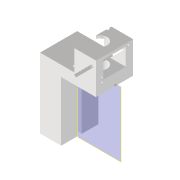
# Autodesk Inventor part: 30_XYTabel_Aliexpress_cellSTORM_lasermount
Saved by Autodesk Inventor 2022 (Build 260153000, 153)
## iProperties
Created: 2021-12-30
Part Number: 30_XYTabel_Aliexpress_cellSTORM_lasermount
Material: Generisch
Document SubType Name: Modeling
Designer: diederichbenedict
Density: 1 g/cm^3
Appearance: Vorgabe
Author: diederichbenedict
Autodesk Inventor part; units mm, degrees
ref_plane "YZ Plane" through (0, 0, 0) normal (1, 0, 0) x (0, 1, 0)
ref_plane "XZ Plane" through (0, 0, 0) normal (0, 1, 0) x (-1, 0, 0)
ref_plane "XY Plane" through (0, 0, 0) normal (0, 0, 1) x (1, 0, 0)
ref_plane "Arbeitsebene1" through (-8.5351, 221.2503, 0) normal (0, 0, -1) x (0, 1, 0)
sketch "Skizze1" plane through (-8.5351, 221.2503, 0) normal (0, 0, -1) x (0, 1, 0)
  circle A0 centre (33, 16) radius 1.4 projected
  circle A1 centre (33, 8) radius 1.4 projected
  circle A2 centre (33, 24) radius 1.4 projected
  circle A3 centre (5, 16) radius 1.4 projected
  circle A4 centre (5, 8) radius 1.4 projected
  circle A5 centre (5, 24) radius 1.4 projected
  circle A6 centre (43, 8) radius 1.4 projected
  circle A7 centre (43, 16) radius 1.4 projected
  circle A8 centre (43, 24) radius 1.4 projected
  line L0 (0, 32) -> (0, 0) projected
  line L1 (0, 32) -> (48, 32) projected
  line L2 (48, 0) -> (48, 32) projected
  line L3 (0, 0) -> (48, 0) projected
  arc A9 (65.2166, -9.3098) -> (65.4479, -9.4649) centre (65.4479, -9.2149) ccw projected
  arc A10 (65.2166, -9.3098) -> (64.7173, -8.7321) centre (64.1062, -9.7649) ccw projected
  arc A11 (64.5955, -8.5388) -> (64.7173, -8.7321) centre (64.8445, -8.517) ccw projected
  line L4 (64.5955, -8.5388) -> (64.5653, -8.1931) projected
  arc A12 (64.5653, -8.1931) -> (64.3162, -7.9649) centre (64.3162, -8.2149) ccw projected
  line L5 (64.3162, -7.9649) -> (63.8638, -7.9649) projected
  arc A13 (63.8638, -7.9649) -> (63.6147, -8.1931) centre (63.8638, -8.2149) ccw projected
  line L6 (63.6147, -8.1931) -> (63.5827, -8.5597) projected
  arc A14 (63.4668, -8.7495) -> (63.5827, -8.5597) centre (63.3336, -8.5379) ccw projected
  arc A15 (63.4668, -8.7495) -> (62.9959, -9.3098) centre (64.1062, -9.7649) ccw projected
  arc A16 (62.7646, -9.4649) -> (62.9959, -9.3098) centre (62.7646, -9.2149) ccw projected
  line L7 (62.7646, -9.4649) -> (62.09, -9.4649) projected
  line L8 (62.09, -9.4649) -> (61.59, -8.9649) projected
  line L9 (61.59, -8.9649) -> (61.59, 2.0351) projected
  line L10 (61.59, 2.0351) -> (62.09, 2.5351) projected
  line L11 (62.09, 2.5351) -> (62.7646, 2.5351) projected
  arc A17 (62.9959, 2.3799) -> (62.7646, 2.5351) centre (62.7646, 2.2851) ccw projected
  arc A18 (62.9959, 2.3799) -> (63.4668, 1.8196) centre (64.1062, 2.8351) ccw projected
  arc A19 (63.5827, 1.6298) -> (63.4668, 1.8196) centre (63.3336, 1.608) ccw projected
  line L12 (63.5827, 1.6298) -> (63.6147, 1.2633) projected
  arc A20 (63.6147, 1.2633) -> (63.8638, 1.0351) centre (63.8638, 1.2851) ccw projected
  line L13 (63.8638, 1.0351) -> (64.3162, 1.0351) projected
  arc A21 (64.3162, 1.0351) -> (64.5653, 1.2633) centre (64.3162, 1.2851) ccw projected
  line L14 (64.5653, 1.2633) -> (64.5955, 1.6089) projected
  arc A22 (64.7173, 1.8023) -> (64.5955, 1.6089) centre (64.8445, 1.5871) ccw projected
  arc A23 (64.7173, 1.8023) -> (65.2166, 2.3799) centre (64.1062, 2.8351) ccw projected
  arc A24 (65.4479, 2.5351) -> (65.2166, 2.3799) centre (65.4479, 2.2851) ccw projected
  line L15 (65.4479, 2.5351) -> (66.59, 2.5351) projected
  line L16 (66.59, 2.5351) -> (66.59, 9.1351) projected
  line L17 (66.59, 9.1351) -> (65.99, 9.7351) projected
  line L18 (65.99, 9.7351) -> (58.19, 9.7351) projected
  line L19 (58.19, 9.7351) -> (56.99, 8.5351) projected
  line L20 (56.99, 8.5351) -> (56.99, -15.4649) projected
  line L21 (56.99, -15.4649) -> (58.19, -16.6649) projected
  line L22 (58.19, -16.6649) -> (65.99, -16.6649) projected
  line L23 (65.99, -16.6649) -> (66.59, -16.0649) projected
  line L24 (66.59, -16.0649) -> (66.59, -9.4649) projected
  line L25 (66.59, -9.4649) -> (65.4479, -9.4649) projected
  circle A25 centre (59.585, 3.4351) radius 2.1 projected
  circle A26 centre (59.585, -10.3649) radius 2.1 projected
  line L26 (56.59, 2.9351) -> (56.59, 9.435) projected
  line L27 (56.99, 2.5351) -> (56.59, 2.9351) projected
  arc A27 (64.7172, 1.8023) -> (65.2166, 2.3799) centre (64.1062, 2.8351) ccw projected
  arc A28 (65.4479, 2.5351) -> (65.2166, 2.3799) centre (65.4479, 2.2851) ccw projected
  line L28 (66.59, 2.5351) -> (65.4479, 2.5351) projected
  line L29 (66.59, 9.4351) -> (66.59, 2.5351) projected
  line L30 (65.99, 10.0351) -> (66.59, 9.4351) projected
  line L31 (57.19, 10.0351) -> (65.99, 10.0351) projected
  line L32 (56.59, 9.435) -> (57.19, 10.0351) projected
  line L33 (56.59, 2.9351) -> (56.59, 9.435) projected
  line L34 (56.99, 2.5351) -> (56.59, 2.9351) projected
  line L35 (56.99, -9.4649) -> (56.99, 2.5351) projected
  line L36 (56.59, -9.8649) -> (56.99, -9.4649) projected
  line L37 (56.59, -16.3649) -> (56.59, -9.8649) projected
  line L38 (57.19, -16.9649) -> (56.59, -16.3649) projected
  line L39 (61.79, -16.9649) -> (57.19, -16.9649) projected
  arc A29 (62.59, -16.9649) -> (61.79, -16.9649) centre (62.19, -17.2649) ccw projected
  line L40 (65.99, -16.9649) -> (62.59, -16.9649) projected
  line L41 (66.59, -16.3649) -> (65.99, -16.9649) projected
  line L42 (66.59, -9.4649) -> (66.59, -16.3649) projected
  line L43 (65.4479, -9.4649) -> (66.59, -9.4649) projected
  arc A30 (65.2166, -9.3098) -> (65.4479, -9.4649) centre (65.4479, -9.2149) ccw projected
  arc A31 (65.2166, -9.3098) -> (64.7172, -8.7321) centre (64.1062, -9.7649) ccw projected
  arc A32 (64.5955, -8.5388) -> (64.7172, -8.7321) centre (64.8445, -8.517) ccw projected
  line L44 (64.5653, -8.1931) -> (64.5955, -8.5388) projected
  arc A33 (64.5653, -8.1931) -> (64.3162, -7.9649) centre (64.3162, -8.2149) ccw projected
  line L45 (63.8638, -7.9649) -> (64.3162, -7.9649) projected
  arc A34 (63.8638, -7.9649) -> (63.6147, -8.1931) centre (63.8638, -8.2149) ccw projected
  line L46 (63.5827, -8.5597) -> (63.6147, -8.1931) projected
  arc A35 (63.4668, -8.7495) -> (63.5827, -8.5597) centre (63.3336, -8.5379) ccw projected
  arc A36 (63.4668, -8.7495) -> (62.9959, -9.3098) centre (64.1062, -9.7649) ccw projected
  arc A37 (62.7646, -9.4649) -> (62.9959, -9.3098) centre (62.7646, -9.2149) ccw projected
  line L47 (62.09, -9.4649) -> (62.7646, -9.4649) projected
  line L48 (61.59, -8.9649) -> (62.09, -9.4649) projected
  line L49 (61.59, 2.0351) -> (61.59, -8.9649) projected
  line L50 (62.09, 2.5351) -> (61.59, 2.0351) projected
  line L51 (62.7646, 2.5351) -> (62.09, 2.5351) projected
  arc A38 (62.9959, 2.3799) -> (62.7646, 2.5351) centre (62.7646, 2.2851) ccw projected
  arc A39 (62.9959, 2.3799) -> (63.4668, 1.8196) centre (64.1062, 2.8351) ccw projected
  arc A40 (63.5827, 1.6298) -> (63.4668, 1.8196) centre (63.3336, 1.6081) ccw projected
  line L52 (63.6147, 1.2633) -> (63.5827, 1.6298) projected
  arc A41 (63.6147, 1.2633) -> (63.8638, 1.0351) centre (63.8638, 1.2851) ccw projected
  line L53 (64.3162, 1.0351) -> (63.8638, 1.0351) projected
  arc A42 (64.3162, 1.0351) -> (64.5653, 1.2633) centre (64.3162, 1.2851) ccw projected
  line L54 (64.5955, 1.6089) -> (64.5653, 1.2633) projected
  arc A43 (64.7172, 1.8023) -> (64.5955, 1.6089) centre (64.8445, 1.5871) ccw projected
  line L55 (85.0966, 28.1351) -> (41.8486, 28.1351)
  line L56 (61.6219, 29.1351) -> (61.6219, 34.6351)
  line L57 (66.9191, 29.1351) -> (66.9191, 34.6351)
  line L58 (0, 0) -> (56.64, 0)
  line L59 (56.64, 0) -> (56.64, -17.0149)
  line L60 (56.64, -17.0149) -> (0, -17.0149)
  line L61 (0, -17.0149) -> (0, 0)
  line L62 (56.64, 0) -> (48, 0)
  line L63 (48, 0) -> (48, 28.1351)
  line L64 (48, 28.1351) -> (56.64, 28.1351)
  line L65 (56.64, 28.1351) -> (56.64, 0)
  line L66 (73.5914, 28.1351) -> (56.64, 28.1351)
  line L67 (56.64, 28.1351) -> (56.64, 10.5351)
  line L68 (56.64, 10.5351) -> (73.5914, 10.5351)
  line L69 (73.5914, 10.5351) -> (73.5914, 28.1351)
  line L70 (73.59, 15.5051) -> (73.59, -22.4349)
  line L71 (73.59, 15.5051) -> (73.59, -22.4349)
  point P0 (-221.2503, 8.5351)
  point P1 (56.64, -16.4149)
  point P2 (56.64, -9.8149)
  point P3 (56.64, 2.8851)
  point P4 (56.64, 9.4851)
  dimension "d0" = 0.5
  constraints: 34 end point, 6 parallel, 4 horizontal, 4 vertical, 3 perpendicular, 3 point on line, 10 other
  measures "d0" distance between parallel lines of L68 L31
extrude "Extrusion1" add sketch "Skizze1" along normal mid plane 30 contours L3 L58 L59 L36 L37 L38 L60 L61 | L2 L55 L65 L32 L26 L27 L58 | L55 L69 L68 L65
sketch "Skizze2" plane through (-25.55, 221.2503, -15) normal (-1, 0, 0) x (0, 0, 1)
  circle A0 centre (15, 5) radius 1.4 projected
  circle A1 centre (15, 33) radius 1.4 projected
  line L0 (15, 33) -> (15, 0) construction
  line L1 (30, 0) -> (0, 0) projected
  line L2 (13.4, 33) -> (13.4, 0)
  line L3 (16.6, 0) -> (16.6, 33)
  arc A2 (16.6, 33) -> (13.4, 33) centre (15, 33) ccw
  arc A3 (13.4, 0) -> (16.6, 0) centre (15, 0) ccw
  point P0 (15, -221.2503)
  point P1 (15, 16.5)
  dimension "d3" = 3.2
  constraints: 8 end point, 4 point on circle, 4 tangent, 2 centre point, 2 midpoint, 1 parallel
  measures "d3" diameter of A3
extrude "Extrusion2" cut sketch "Skizze2" against normal blind 30 contours A0 | A1 | A3 L1 | L1 L2 A2 L3
sketch "Skizze3" plane through (19.6, 269.2503, -15) normal (1, 0, 0) x (0, 0, -1)
  arc A0 (0.8555, 0.89) -> (1.8555, -0.11) centre (1.8555, 0.89) ccw projected
  line L0 (1.8555, -0.11) -> (5, -0.11) projected
  line L1 (5, -0.11) -> (5, 25.59) projected
  line L2 (5, 25.59) -> (-4.5277, 25.59) projected
  arc A1 (-4.5277, 25.59) -> (-5.5277, 24.59) centre (-4.5277, 24.59) ccw projected
  line L3 (-5.5277, 24.59) -> (-5.5277, 22.7276) projected
  arc A2 (-6.5277, 21.7276) -> (-5.5277, 22.7276) centre (-6.5277, 22.7276) ccw projected
  line L4 (-6.5277, 21.7276) -> (-25, 21.7276) projected
  line L5 (-25, 21.7276) -> (-25, 10.193) projected
  arc A3 (-26, 9.193) -> (-25, 10.193) centre (-26, 10.193) ccw projected
  line L6 (-26, 9.193) -> (-27, 9.193) projected
  arc A4 (-27, 9.193) -> (-28, 8.193) centre (-27, 8.193) ccw projected
  line L7 (-28, 8.193) -> (-28, 5.6276) projected
  arc A5 (-28, 5.6276) -> (-27, 4.6276) centre (-27, 5.6276) ccw projected
  line L8 (-27, 4.6276) -> (-0.1445, 4.6276) projected
  arc A6 (0.8555, 3.6276) -> (-0.1445, 4.6276) centre (-0.1445, 3.6276) ccw projected
  line L9 (0.8555, 3.6276) -> (0.8555, 0.89) projected
  line L10 (-7.5, 6.59) -> (-23, 6.59) projected
  line L11 (-23, 6.59) -> (-23, 20.09) projected
  line L12 (-23, 20.09) -> (-7.5, 20.09) projected
  line L13 (-7.5, 20.09) -> (-7.5, 6.59) projected
  circle A7 centre (2.5, 2.59) radius 1 projected
  circle A8 centre (-4, 23.09) radius 1 projected
  circle A9 centre (-25.5, 7.59) radius 1 projected
  point P0 (-15, -269.2503)
  point P1 (2.5, 6.2705)
  point P2 (-4, 26.7705)
  point P3 (-25.5, 11.2705)
hole "Bohrung1" at (19.6, 275.5208, -17.5) at (19.6, 296.0208, -11) at (19.6, 276.8403, 10.5) at (19.6, 280.5208, 10.5) at (19.6, 292.3403, -11) direction (-1, 0, 0) diameter 1.7 end through all
sketch "Skizze4" plane through (19.6, 269.2503, -15) normal (1, 0, 0) x (0, 0, -1)
  circle A0 centre (-15, 16.2705) radius 2.6486 projected
  line L0 (-6, 9.2705) -> (-24, 9.2705)
  line L1 (-24, 9.2705) -> (-24, 23.2705)
  line L2 (-24, 23.2705) -> (-6, 23.2705)
  line L3 (-6, 23.2705) -> (-6, 9.2705)
  line L4 (-6, 9.2705) -> (-24, 23.2705) construction
  line L5 (-24, 9.2705) -> (-6, 23.2705) construction
  point P0 (-15, -269.2503)
  dimension "d13" = 18
  dimension "d14" = 14
  constraints: 12 end point, 2 midpoint, 2 parallel, 1 horizontal, 1 perpendicular
  measures "d13" distance of L1.end L2.end
  measures "d14" distance of L0.end L1.end
extrude "Extrusion3" cut sketch "Skizze4" against normal blind 30 contours A0 | L0 L1 L2 L3
sketch "Skizze5" plane through (2, 294.8418, -15) normal (0, 1, 0) x (1, 0, 0)
  circle A0 centre (5.4649, -15) radius 6 projected
  point P0 (-2, -15)
extrude "Extrusion4" cut sketch "Skizze5" against normal blind 30
sketch "Skizze6" plane through (-8.5351, 221.2503, -15) normal (0, 0, -1) x (-1, 0, 0)
  line L0 (-13.5, 41.6) -> (-13.5, 0)
  line L1 (-18.5, 41.6) -> (-18.5, 0)
  line L2 (-29.1351, 68.7705) -> (-34.6351, 68.7705) projected
  line L3 (-29.1351, 66.9191) -> (-34.6351, 66.9191)
  line L4 (-29.1351, 61.6219) -> (-34.6351, 61.6219)
  line L5 (-10, 48) -> (-22, 48) projected
  line L6 (-16, 48) -> (-16, 67.9487)
  line L7 (-24.6296, 69.2196) -> (-10.4875, 55.0775)
  line L8 (-10.4875, 55.0775) -> (-11.9017, 53.6633)
  line L9 (-11.9017, 53.6633) -> (-26.0438, 67.8054)
  line L10 (-26.0438, 67.8054) -> (-24.6296, 69.2196)
  line L11 (-24.6296, 69.2196) -> (-11.9017, 53.6633) construction
  line L12 (-10.4875, 55.0775) -> (-26.0438, 67.8054) construction
  line L13 (-24.6296, 69.2196) -> (-4.6296, 69.2196) construction
  line L14 (-28.0351, 60.59) -> (-35.7351, 60.59)
  line L15 (-29.1351, 57.9414) -> (-34.6351, 57.9414)
  line L16 (-29.1351, 63.2386) -> (-34.6351, 63.2386)
  line L17 (-28.0351, 60.59) -> (-35.7351, 60.59)
  line L18 (-35.7351, 60.59) -> (-16, 60.59)
  point P0 (-8.5351, -221.2503)
  point P1 (-18.2657, 61.4415)
  point P2 (-16, 60.5193)
  dimension "d19" = 5.2972
  dimension "d21" = 20
  dimension "d22" = 45
  dimension "d23" = 2
  dimension "d42" = 0.05
  constraints: 34 end point, 7 horizontal, 4 point on line, 3 midpoint, 3 vertical, 2 parallel, 1 equal length, 1 perpendicular, 16 other
  measures "d19" distance between parallel lines of L4 L3
  measures "d21" distance of L7.start L7.end
  measures "d22" angle of L7 L13
  measures "d23" distance of L7.end L8.end
  measures "d42" distance from line of point (-16, 60.519) L7
extrude "Extrusion5" cut sketch "Skizze6" against normal blind 30
sketch "Skizze7" plane through (-25.55, 221.2503, 15) normal (0, -1, 0) x (1, 0, 0)
  circle A0 centre (3.55, -25) radius 1.75 projected
  circle A1 centre (3.55, -5) radius 1.75 projected
  circle A2 centre (23.55, -5) radius 1.75 projected
  circle A3 centre (23.55, -25) radius 1.75 projected
  point P0 (25.55, -15)
hole "Bohrung2" at (-2, 221.2503, -10) at (-2, 221.2503, 10) direction (0, 1, 0) diameter 3 end through all counterbore diameter 6.5 counterbore depth 50
sketch "Skizze8" plane through (3.3666, 274.9136, 4.3822) normal (-0.7071, 0.7071, 0) x (-0.7071, -0.7071, 0)
  ellipse E0 centre (-5.7959, -4.3822) end of major axis (-14.2811, -4.3822) minor radius 6 (-5.1013, -10.3621) -> (0, -8.7645) ccw projected
  line L0 (-5.1013, -13.3822) -> (-5.1013, -10.3621) projected
  line L1 (-20, -13.3822) -> (-5.1013, -13.3822) projected
  line L2 (-20, -19.3822) -> (-20, -13.3822) projected
  line L3 (0, -19.3822) -> (-20, -19.3822) projected
  line L4 (0, -19.3822) -> (0, -8.7645) projected
  ellipse E1 centre (-7.9298, 6.1178) end of major axis (-9.1319, 6.1178) minor radius 0.85 projected
  ellipse E2 centre (-5.7959, -4.3822) end of major axis (-14.2811, -4.3822) minor radius 6 (0, 0) -> (-5.1013, 1.5976) ccw projected
  line L5 (0, 0) -> (0, 10.6178) projected
  line L6 (-20, 10.6178) -> (0, 10.6178) projected
  line L7 (-20, 4.6178) -> (-20, 10.6178) projected
  line L8 (-5.1013, 4.6178) -> (-20, 4.6178) projected
  line L9 (-5.1013, 1.5976) -> (-5.1013, 4.6178) projected
  circle A0 centre (-12.5507, 7.6178) radius 1.4
  circle A1 centre (-12.5507, -16.3822) radius 1.4
  line L10 (-5.1013, -13.3822) -> (-5.1013, -10.3621) projected
  line L11 (-20, -13.3822) -> (-5.1013, -13.3822) projected
  line L12 (0, -19.3822) -> (-20, -19.3822) projected
  line L13 (-5.1013, 4.6178) -> (-20, 4.6178) projected
  line L14 (-5.1013, 1.5976) -> (-5.1013, 4.6178) projected
  line L15 (-20, 10.6178) -> (0, 10.6178) projected
  ellipse E3 centre (-5.7959, -4.3822) end of major axis (-14.2811, -4.3822) minor radius 6 (-5.1013, -10.3621) -> (0, -8.7645) ccw projected
  line L16 (-20, -19.3822) -> (-20, -13.3822) projected
  line L17 (0, -19.3822) -> (0, -8.7645) projected
  ellipse E4 centre (-5.7959, -4.3822) end of major axis (-14.2811, -4.3822) minor radius 6 (0, 0) -> (-5.1013, 1.5976) ccw projected
  line L18 (0, 0) -> (0, 10.6178) projected
  line L19 (-20, 4.6178) -> (-20, 10.6178) projected
  ellipse E5 centre (-2.7248, 6.1178) end of major axis (-3.9269, 6.1178) minor radius 0.85 projected
  ellipse E6 centre (-2.7248, 6.1178) end of major axis (-3.9269, 6.1178) minor radius 0.85 projected
  point P0 (196.7739, -4.3822)
  dimension "d33" = 2.8
  dimension "d34" = 2.8
  constraints: 2 centre point, 7 other
  measures "d33" diameter of A0
  measures "d34" diameter of A1
hole "Bohrung3" at (12.2413, 283.7883, 12) at (12.2413, 283.7883, -12) direction (-0.7071, 0.7071, 0) diameter 2.8 end through all
sketch "Skizze10" plane through (-25.55, 221.2503, 15) normal (0, -1, 0) x (1, 0, 0)
  line L0 (17.0149, -16.6) -> (0, -16.6) projected
  line L1 (0, -30) -> (0, -16.6) projected
  line L2 (17.0149, -30) -> (0, -30) projected
  line L3 (17.0149, -16.6) -> (17.0149, -30) projected
  line L4 (0.65, 1.2) -> (0.65, -31.2) projected
  line L5 (0, -13.4) -> (17.0149, -13.4) projected
  line L6 (17.0149, 0) -> (17.0149, -13.4) projected
  line L7 (0, 0) -> (17.0149, 0) projected
  line L8 (0, -13.4) -> (0, 0) projected
  line L9 (-3.85, -11.5) -> (5.15, -11.5)
  line L10 (5.15, -11.5) -> (5.15, -18.5)
  line L11 (5.15, -18.5) -> (-3.85, -18.5)
  line L12 (-3.85, -18.5) -> (-3.85, -11.5)
  line L13 (-3.85, -11.5) -> (5.15, -18.5) construction
  line L14 (5.15, -11.5) -> (-3.85, -18.5) construction
  point P0 (25.55, -15)
  point P1 (0.65, -15)
  dimension "d46" = 9
  dimension "d47" = 7
  constraints: 12 end point, 3 midpoint, 2 parallel, 1 horizontal, 1 perpendicular
  measures "d46" distance of L10.end L11.end
  measures "d47" distance of L9.end L10.end
extrude "Extrusion7" cut sketch "Skizze10" against normal blind 35 contours L10 L11 L4 L0 | L0 L4 L5 L10 | L4 L11 L1 L0 | L0 L1 L11 L12 L9 L8 L5 L4 | L5 L4 L9 L10 | L5 L8 L9 L4
sketch "Skizze11" plane through (-25.55, 221.2503, 15) normal (-1, 0, 0) x (0, 0, 1)
  circle A0 centre (-47.5, 46.7901) radius 1.4 projected
  circle A1 centre (-25.2207, 46.7901) radius 1.4
  point P0 (-15, -221.2503)
  dimension "d50" = 2.8
  constraints: 1 centre point
  measures "d50" diameter of A1
extrude "Extrusion8" cut sketch "Skizze11" against normal blind 15 contours A1
